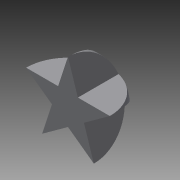
# Autodesk Inventor part: star
Saved by Autodesk Inventor 2013 (Build 170138000, 138)
## iProperties
Created: 2014-05-08
Part Number: star
Material: 一般
Document SubType Name: Modeling
Designer: andou
Density: 1 g/cm^3
Author: andou
Autodesk Inventor part; units mm, degrees
ref_plane "YZ Plane" through (0, 0, 0) normal (1, 0, 0) x (0, 1, 0)
ref_plane "XZ Plane" through (0, 0, 0) normal (0, 1, 0) x (-1, 0, 0)
ref_plane "XY Plane" through (0, 0, 0) normal (0, 0, 1) x (1, 0, 0)
sketch "スケッチ1" plane through (0, 0, 0) normal (0, 0, 1) x (1, 0, 0)
  arc A0 (5, 0) -> (0, 5) centre (0, 0) ccw
  line L0 (0, 0) -> (5, 0)
  line L1 (0, 5) -> (0, 0)
  point P0 (0, 0)
  dimension "d0" = 10
  constraints: 4 end point, 2 point on circle, 1 centre point, 1 coincident, 1 horizontal, 1 perpendicular
  measures "d0" diameter of A0
revolve "回転1" add sketch "スケッチ1" angle 360 about axis through (0, 5, 0) along (0, -1, 0)
sketch "スケッチ2" plane through (0, 0, 0) normal (0, -1, 0) x (1, 0, 0)
  circle A0 centre (0, 0) radius 5 projected
  line L0 (0, 5) -> (-1.1226, 1.5451)
  line L1 (-4.7553, 1.5451) -> (-1.8164, -0.5902)
  line L2 (-1.8164, -0.5902) -> (-2.9389, -4.0451)
  line L3 (-2.9389, -4.0451) -> (0, -1.9098)
  line L4 (0, -1.9098) -> (2.9389, -4.0451)
  line L5 (2.9389, -4.0451) -> (1.8164, -0.5902)
  line L6 (1.8164, -0.5902) -> (4.7553, 1.5451)
  line L7 (4.7553, 1.5451) -> (1.1226, 1.5451)
  line L8 (1.1226, 1.5451) -> (0, 5)
  line L9 (0, 5) -> (-1.1226, 1.5451)
  line L10 (1.1226, 1.5451) -> (4.7553, 1.5451)
  line L11 (4.7553, 1.5451) -> (1.8164, -0.5902)
  line L12 (1.8164, -0.5902) -> (2.9389, -4.0451)
  line L13 (2.9389, -4.0451) -> (0, -1.9098)
  line L14 (2.9389, -4.0451) -> (0, -1.9098)
  line L15 (-1.8164, -0.5902) -> (-4.7553, 1.5451)
  line L16 (4.7553, 1.5451) -> (1.8164, -0.5902)
  line L17 (0, -1.9098) -> (-2.9389, -4.0451)
  line L18 (-4.7553, 1.5451) -> (-1.1226, 1.5451)
  line L19 (1.1226, 1.5451) -> (4.7553, 1.5451)
  line L20 (0, 5) -> (-1.1226, 1.5451)
  line L21 (-1.8164, -0.5902) -> (-2.9389, -4.0451)
  line L22 (2.9389, -4.0451) -> (1.8164, -0.5902)
  line L23 (1.1226, 1.5451) -> (0, 5)
  constraints: 48 end point, 9 collinear, 1 coincident, 1 vertical alignment, 7 other
extrude "押し出し1" cut sketch "スケッチ2" against normal blind 10 contours L6 L5 L4 L3 L2 L1 L18 L0 L8 L7 keep common part
